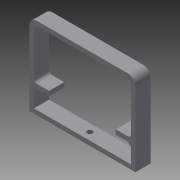
# Autodesk Inventor part: dcdcSupport
Saved by Autodesk Inventor 2014 SP2 (Build 180246200, 246)
## iProperties
Created: 2020-05-14
Part Number: dcdcSupport
Material: Generic
Document SubType Name: Sheet Metal
Designer: GauchoHP
Density: 1 g/cm^3
Sheet Metal Rule: Default_mm
Appearance: Default
Author: GauchoHP
Autodesk Inventor part; units mm, degrees
ref_plane "YZ Plane" through (0, 0, 0) normal (1, 0, 0) x (0, 1, 0)
ref_plane "XZ Plane" through (0, 0, 0) normal (0, 1, 0) x (-1, 0, 0)
ref_plane "XY Plane" through (0, 0, 0) normal (0, 0, 1) x (1, 0, 0)
sketch "Sketch1" plane through (0, 0, 0) normal (0, 1, 0) x (-1, 0, 0)
  line L0 (-30, 16.5) -> (30, 16.5)
  line L1 (32, 14.5) -> (32, -14.5)
  line L2 (-32, -14.5) -> (-32, 14.5)
  arc A0 (-32, -14.5) -> (-30, -16.5) centre (-30, -14.5) ccw
  arc A1 (-30, 16.5) -> (-32, 14.5) centre (-30, 14.5) ccw
  arc A2 (32, 14.5) -> (30, 16.5) centre (30, 14.5) ccw
  arc A3 (30, -16.5) -> (32, -14.5) centre (30, -14.5) ccw
  line L3 (-35, 14.5) -> (-35, -34.5)
  line L4 (35, -34.5) -> (35, 14.5)
  arc A4 (35, 14.5) -> (30, 19.5) centre (30, 14.5) ccw
  line L5 (30, 19.5) -> (-30, 19.5)
  arc A5 (-30, 19.5) -> (-35, 14.5) centre (-30, 14.5) ccw
  line L6 (35, -34.5) -> (-35, -34.5)
  line L7 (-22, -16.5) -> (-22, -19.5)
  line L8 (22, -16.5) -> (22, -19.5)
  line L9 (30, -16.5) -> (22, -16.5)
  line L10 (-22, -16.5) -> (-30, -16.5)
  line L11 (-30, -19.5) -> (-22, -19.5)
  line L12 (22, -19.5) -> (30, -19.5)
  line L13 (32, -31.5) -> (-32, -31.5)
  line L14 (-32, -31.5) -> (-32, -21.5)
  line L15 (-32, -14.5) -> (-32, 14.5)
  line L16 (32, 14.5) -> (32, -14.5)
  line L17 (32, -21.5) -> (32, -31.5)
  line L18 (-30, -19.5) -> (-32, -21.5)
  line L19 (32, -21.5) -> (30, -19.5)
  point P0 (0, 0)
  point P1 (32, -16.5)
  point P2 (32, 16.5)
  point P3 (-32, -16.5)
  point P4 (-32, -19.5)
  point P5 (32, -19.5)
  dimension "d0" = 64
  dimension "d1" = 33
  dimension "d2" = 32
  dimension "d3" = 16.5
  dimension "d4" = 2
  dimension "d5" = 3
  dimension "d6" = 70
  dimension "d9" = 10
  dimension "d10" = 10
  dimension "d11" = 20
  dimension "d12" = 3
  dimension "d13" = 2
  dimension "d14" = 2
  dimension "d15" = 2
  dimension "d16" = 2
  constraints: 40 end point, 12 point on circle, 10 parallel, 10 tangent, 8 point on line, 6 centre point, 6 perpendicular, 3 equal radius, 1 horizontal, 2 other
  measures "d0" distance of point (32, -16.5) point (-32, -16.5)
  measures "d1" distance of point (32, 16.5) point (32, -16.5)
  measures "d2" distance from line of L2 point (0, 0)
  measures "d3" distance from line of L0 point (0, 0)
  measures "d4" radius of A0
  measures "d5" distance between parallel lines of L3 L2
  measures "d6" distance of L4.start L3.end
  measures "d9" distance between parallel lines of L7 L2
  measures "d10" distance between parallel lines of L8 L1
  measures "d11" distance from line of A0.centre L6
  measures "d12" distance between parallel lines of L6 L13
  measures "d13" distance of L11.start point (-32, -19.5)
  measures "d14" distance of L14.end point (-32, -19.5)
  measures "d15" distance of L17.start point (32, -19.5)
  measures "d16" distance of L12.end point (32, -19.5)
extrude "Extrusion1" add sketch "Sketch1" along normal blind 10
sketch "Sketch2" plane through (35, 0, -34.5) normal (0, 0, -1) x (-1, 0, 0)
  line L0 (0, 10) -> (70, 0)
  line L1 (70, 10) -> (0, 0)
  circle A0 centre (35, 5) radius 1.75
  point P0 (35, 0)
  dimension "d19" = 3.5
  constraints: 4 end point, 1 centre point, 1 midpoint
  measures "d19" diameter of A0
extrude "Extrusion2" cut sketch "Sketch2" against normal blind 10
equation "\"d14\" = d13"
equation "\"d15\" = d13"
equation "\"d16\" = d15"
equation "\"BendRadius\" = Thickness"
equation "\"BendReliefWidth\" = Thickness"
equation "\"BendReliefDepth\" = 0.5 * Thickness"
equation "\"CornerReliefSize\" = 4 * Thickness"
equation "\"MinimumRemnant\" = 2 * Thickness"
equation "\"TransitionRadius\" = BendRadius"
equation "\"JacobiRadiusSize\" = BendRadius"
equation "\"GapSize\" = Thickness"
equation "\"Thickness\" = 0.5"
body "Solid1"
